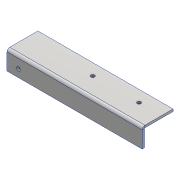
# Autodesk Inventor part: endcapOptionLeftAngle
Saved by Autodesk Inventor 2016 (Build 200138000, 138)
## iProperties
Created: 2015-05-12
Part Number: endcapOptionLeftAngle
Material: Aluminum 6061
Document SubType Name: Sheet Metal
Designer: krosie
Density: 2.7 g/cm^3
Sheet Metal Rule: Aluminium
Appearance: Aluminum - Flat
Flat Pattern Width: 6.08588 cm
Flat Pattern Length: 17.5 cm
Flat Pattern Area: 106.503 cm^2
Sheet Metal Width: 60.859 mm
Sheet Metal Length: 175.000 mm
Sheet Metal Area: 10650.299 mm^2
Author: krosie
Autodesk Inventor part; units mm, degrees
ref_plane "YZ Plane" through (0, 0, 0) normal (1, 0, 0) x (0, 1, 0)
ref_plane "XZ Plane" through (0, 0, 0) normal (0, 1, 0) x (-1, 0, 0)
ref_plane "XY Plane" through (0, 0, 0) normal (0, 0, 1) x (1, 0, 0)
sketch "Sketch1" plane through (0, 0, 0) normal (0, 0, 1) x (1, 0, 0)
  line L0 (0, 0) -> (175, 0)
  line L1 (175, 0) -> (175, 40)
  line L2 (175, 40) -> (0, 40)
  line L3 (0, 40) -> (0, 0)
  dimension "d0" = 175
  dimension "d1" = 40
  measures "d0" distance of L0.start L0.end
  measures "d1" distance of L0.end L1.end
extrude "Plate1" add sketch "Sketch1" along normal blind 3
sketch "Sketch2" plane through (0, 3, 3) normal (0, -1, 0) x (1, 0, 0)
  line L0 (175, 0) -> (0, 0)
  line L1 (0, 0) -> (0, -25)
  line L2 (0, -25) -> (175, -25)
  line L3 (175, -25) -> (175, 0)
  constraints: 6 end point, 1 horizontal, 1 perpendicular, 1 vertical
edge flange "Flange1" height 25 angle 90 thickness 3 bend radius 0.5 thickness toward (0, -1, 0) relief tear relief width 3 relief depth 1.5 edges at (87.5, 0, 0) wall of the first edge with corners at (175, 3, 3) (0, 3, 3) (0, 3, -22) (175, 3, -22)
bend "Bend1"
corner "Corner1"
hole "Hole3" at (146, 25, 3) direction (0, 0, -1) diameter 5 end through all
hole "Hole4" at (86, 25, 3) direction (0, 0, -1) diameter 5 end through all
hole "Hole5" at (15, 3, -12) direction (0, -1, 0) diameter 5 end through all
equation "\"d38\" = Thickness"
equation "\"d47\" = Thickness"
equation "\"d56\" = Thickness"
equation "\"d3\" = BendReliefWidth"
equation "\"d4\" = BendReliefDepth"
equation "\"d5\" = MinimumRemnant"
equation "\"d6\" = BendRadius"
equation "\"d10\" = CornerReliefSize"
equation "\"d11\" = GapSize"
equation "\"d12\" = JacobiRadiusSize"
equation "\"BendRadius\" = Thickness"
equation "\"BendReliefWidth\" = Thickness"
equation "\"BendReliefDepth\" = 0.5 * Thickness"
equation "\"CornerReliefSize\" = 4 * Thickness"
equation "\"MinimumRemnant\" = 2 * Thickness"
equation "\"TransitionRadius\" = BendRadius"
equation "\"JacobiRadiusSize\" = BendRadius"
equation "\"GapSize\" = Thickness"
equation "\"d2\" = BendRadius"
equation "\"Thickness\" = 3"
body "Solid1"
